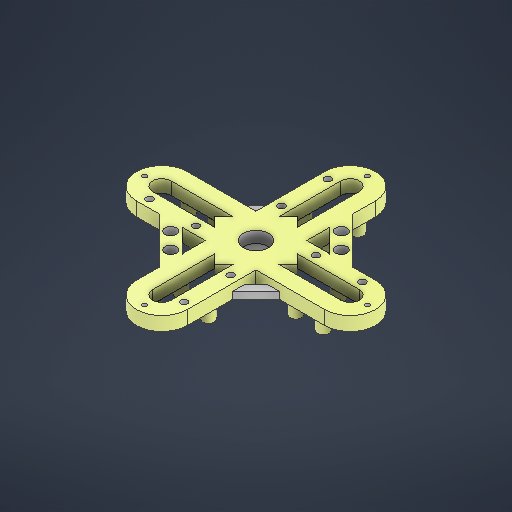
# Autodesk Inventor part: Redesign_Gripper_Baseplate
Saved by Autodesk Inventor 2025.1 (Build 291241000, 241)
## iProperties
Created: 2024-12-19
Part Number: Redesign_Gripper_Baseplate
Material: Generic
Document SubType Name: Modeling
Designer: m_kni
Density: 1 g/cm^3
Appearance: Default
Finish1_Area: 11299.045 mm^2
Finish1_Appearance: Satin - Lemon Chiffon
Finish1_Process: Prime/Paint RAL 3018
Finish1_Description: Prime/Paint RAL 3018
Finish1_ShortDescription: RAL 3018
Finish1_Thickness: 0.050 mm
Author: m_kni
## iProperties of the stored document Redesign_Gripper_Baseplate_3DPrint.ipt
Created: 2025-01-24
Part Number: Redesign_Gripper_Baseplate_3DPrint
Material: Generic
Document SubType Name: Modeling
Designer: m_kni
Density: 1 g/cm^3
Appearance: Default
Author: m_kni
Autodesk Inventor part; units mm, degrees
ref_plane "YZ Plane" through (0, 0, 0) normal (1, 0, 0) x (0, 1, 0)
ref_plane "XZ Plane" through (0, 0, 0) normal (0, 1, 0) x (-1, 0, 0)
ref_plane "XY Plane" through (0, 0, 0) normal (0, 0, 1) x (1, 0, 0)
sketch "Sketch1" plane through (0, 0, 0) normal (0, 1, 0) x (-1, 0, 0)
  line L0 (17.9605, 0) -> (0, -17.9605)
  line L1 (17.9605, 0) -> (43.3605, 0) construction
  line L2 (17.9605, 0) -> (0, 17.9605)
  line L3 (17.9605, 0) -> (43.3605, 0) construction
  line L4 (-17.9605, 0) -> (0, -17.9605)
  line L5 (-17.9605, 0) -> (0, 17.9605)
  line L6 (0, 15.4205) -> (-15.4205, 0)
  line L7 (0, 15.4205) -> (21.8079, 15.4205) construction
  line L8 (-15.4205, 0) -> (0, -15.4205)
  line L9 (0, -15.4205) -> (15.4205, 0)
  line L10 (15.4205, 0) -> (0, 15.4205)
  line L11 (0, -40.8205) -> (2, -40.8205)
  line L12 (0, -40.8205) -> (-2, -40.8205)
  circle A0 centre (7.5, -28.1205) radius 2.5
  line L13 (4, -28.1205) -> (4, -13.9605)
  line L14 (4, -28.1205) -> (4, -40.8205)
  line L15 (11, -6.9605) -> (11, -40.8205)
  arc A1 (-4, -40.8205) -> (4, -40.8205) centre (0, -40.8205) ccw
  line L16 (0, -15.4205) -> (0, -17.9605)
  line L17 (-4, -40.8205) -> (-4, -13.9605)
  line L18 (-11, -40.8205) -> (-11, -6.9605)
  arc A2 (-11, -40.8205) -> (11, -40.8205) centre (0, -40.8205) ccw
  circle A3 centre (-7.5, -24.8705) radius 2.5
  circle A4 centre (-7.5, -36.6205) radius 2.5
  line L19 (15.4205, 0) -> (17.9605, 0)
  line L20 (28.1205, 4) -> (13.9605, 4)
  circle A5 centre (28.1205, 7.5) radius 2.5
  circle A6 centre (24.8705, -7.5) radius 2.5
  line L21 (6.9605, 11) -> (40.8205, 11)
  line L22 (40.8205, -11) -> (6.9605, -11)
  line L23 (40.8205, -4) -> (13.9605, -4)
  line L24 (28.1205, 4) -> (40.8205, 4)
  line L25 (40.8205, 0) -> (40.8205, 2)
  circle A7 centre (36.6205, -7.5) radius 2.5
  line L26 (40.8205, 0) -> (40.8205, -2)
  arc A8 (40.8205, -4) -> (40.8205, 4) centre (40.8205, 0) ccw
  arc A9 (40.8205, -11) -> (40.8205, 11) centre (40.8205, 0) ccw
  line L27 (0, 15.4205) -> (0, 17.9605)
  line L28 (-4, 28.1205) -> (-4, 13.9605)
  circle A10 centre (-7.5, 28.1205) radius 2.5
  circle A11 centre (7.5, 24.8705) radius 2.5
  line L29 (-11, 6.9605) -> (-11, 40.8205)
  line L30 (11, 40.8205) -> (11, 6.9605)
  line L31 (4, 40.8205) -> (4, 13.9605)
  line L32 (-4, 28.1205) -> (-4, 40.8205)
  line L33 (0, 40.8205) -> (-2, 40.8205)
  circle A12 centre (7.5, 36.6205) radius 2.5
  line L34 (0, 40.8205) -> (2, 40.8205)
  arc A13 (4, 40.8205) -> (-4, 40.8205) centre (0, 40.8205) ccw
  arc A14 (11, 40.8205) -> (-11, 40.8205) centre (0, 40.8205) ccw
  line L35 (-15.4205, 0) -> (-17.9605, 0)
  line L36 (-28.1205, -4) -> (-13.9605, -4)
  circle A15 centre (-28.1205, -7.5) radius 2.5
  circle A16 centre (-24.8705, 7.5) radius 2.5
  line L37 (-6.9605, -11) -> (-40.8205, -11)
  line L38 (-40.8205, 11) -> (-6.9605, 11)
  line L39 (-40.8205, 4) -> (-13.9605, 4)
  line L40 (-28.1205, -4) -> (-40.8205, -4)
  line L41 (-40.8205, 0) -> (-40.8205, -2)
  circle A17 centre (-36.6205, 7.5) radius 2.5
  line L42 (-40.8205, 0) -> (-40.8205, 2)
  arc A18 (-40.8205, 4) -> (-40.8205, -4) centre (-40.8205, 0) ccw
  arc A19 (-40.8205, 11) -> (-40.8205, -11) centre (-40.8205, 0) ccw
  point P0 (0, 0)
  point P1 (0, -28.1205)
  point P2 (2, -28.1205)
  point P3 (-2, -22.1205)
  point P4 (-7.5, -22.1205)
  point P5 (-2, -34.1205)
  point P6 (-7.5, -34.1205)
  point P7 (11, -28.1205)
  point P8 (28.1205, 2)
  point P9 (28.1205, 11)
  point P10 (34.1205, -7.5)
  point P11 (34.1205, -2)
  point P12 (22.1205, -7.5)
  point P13 (22.1205, -2)
  point P14 (28.1205, 0)
  point P15 (-2, 28.1205)
  point P16 (-11, 28.1205)
  point P17 (7.5, 34.1205)
  point P18 (2, 34.1205)
  point P19 (7.5, 22.1205)
  point P20 (2, 22.1205)
  point P21 (0, 28.1205)
  point P22 (-28.1205, -2)
  point P23 (-28.1205, -11)
  point P24 (-34.1205, 7.5)
  point P25 (-34.1205, 2)
  point P26 (-22.1205, 7.5)
  point P27 (-22.1205, 2)
  point P28 (-28.1205, 0)
  point P29 (11, 11)
  point P30 (-11, 11)
  point P31 (-11, -11)
  point P32 (11, -11)
  dimension "d12" = 25.4
  dimension "d15" = 25.4
  dimension "d18" = 2.54
  dimension "d19" = 135
  dimension "d25" = 5
  dimension "d41" = 360
  constraints: 86 end point, 20 centre point, 16 coincident, 16 point on circle, 12 point on line, 5 vertical, 4 parallel, 3 equal length, 3 horizontal, 3 perpendicular, 173 other
  measures "d12" distance of L0.start L0.end
  measures "d15" distance of L0.start L2.end
  measures "d18" distance of L6.start L2.end
  measures "d19" angle of L6 L7
  measures "d25" diameter of A0
extrude "Extrusion1" add sketch "Sketch1" along normal blind 6 contours L19 L10 L27 L2 | L0 L16 L9 L19 | L23 A8 L24 L20 L2 L30 L21 A9 L22 L15 L0 | L9 L8 L6 L10 | L15 L22 L0 | L2 L21 L30 | L16 L4 L35 L8 | L6 L35 L5 L27 | L22 L15 A2 L18 L37 L4 L17 A1 L14 L13 L0 | L2 L31 A13 L32 L28 L5 L38 L29 A14 L30 L21 | L4 L18 L37 A19 L38 L29 L5 L39 A18 L40 L36 | L37 L18 L4 | L5 L29 L38 | A0 | A3 | A4 | A5 | A6 | A7 | A10 | A11 | A12 | A15 | A16 | A17
extrude "Extrusion2" add sketch "Sketch1" against normal blind 5.6 contours A0 | A3 | A4 | A5 | A6 | A7 | A10 | A11 | A12 | A15 | A16 | A17
sketch "Sketch2" plane through (0, 0, 0) normal (0, -1, 0) x (1, 0, 0)
  circle A0 centre (7.5, 28.1205) radius 2.5 projected
  circle A1 centre (7.5, 28.1205) radius 2.625
  circle A2 centre (-7.5, 36.6205) radius 2.5 projected
  circle A3 centre (-7.5, 36.6205) radius 2.625
  circle A4 centre (-7.5, 24.8705) radius 2.5 projected
  circle A5 centre (-7.5, 24.8705) radius 2.625
  circle A6 centre (-28.1205, 7.5) radius 2.625
  circle A7 centre (-36.6205, -7.5) radius 2.625
  circle A8 centre (-24.8705, -7.5) radius 2.625
  circle A9 centre (-7.5, -28.1205) radius 2.625
  circle A10 centre (7.5, -36.6205) radius 2.625
  circle A11 centre (7.5, -24.8705) radius 2.625
  circle A12 centre (28.1205, -7.5) radius 2.625
  circle A13 centre (36.6205, 7.5) radius 2.625
  circle A14 centre (24.8705, 7.5) radius 2.625
  point P0 (0, 0)
  dimension "d47" = 5.25
  dimension "d48" = 5.25
  dimension "d49" = 5.25
  dimension "d52" = 360
  constraints: 12 centre point, 3 coincident, 25 other
  measures "d47" diameter of A1
  measures "d48" diameter of A3
  measures "d49" diameter of A5
extrude "Extrusion3" add sketch "Sketch2" along normal blind 0.6 contours A0 | A1 | A2 | A3 | A4 | A5 | A6 | A7 | A8 | A9 | A10 | A11 | A12 | A13 | A14
sketch "Sketch3" plane through (7.5, -5.6, 28.1205) normal (0, -1, 0) x (1, 0, 0)
  circle A0 centre (0, 0) radius 1
  circle A1 centre (-15, 8.5) radius 2.5 projected
  circle A2 centre (-15, 8.5) radius 1
  circle A3 centre (-15, -3.25) radius 2.5 projected
  circle A4 centre (-15, -3.25) radius 1
  circle A5 centre (-44.1205, -35.6205) radius 1
  circle A6 centre (-32.3705, -35.6205) radius 1
  circle A7 centre (-35.6205, -20.6205) radius 1
  circle A8 centre (0, -64.741) radius 1
  circle A9 centre (0, -52.991) radius 1
  circle A10 centre (-15, -56.241) radius 1
  circle A11 centre (29.1205, -20.6205) radius 1
  circle A12 centre (17.3705, -20.6205) radius 1
  circle A13 centre (20.6205, -35.6205) radius 1
  point P0 (-7.5, -28.1205)
  dimension "d56" = 2
  dimension "d57" = 2
  dimension "d58" = 2
  dimension "d61" = 360
  constraints: 12 centre point, 2 coincident, 25 other
  measures "d56" diameter of A0
  measures "d57" diameter of A2
  measures "d58" diameter of A4
extrude "Extrusion4" cut sketch "Sketch3" against normal blind 6 contours A0 | A2 | A4 | A5 | A6 | A7 | A8 | A9 | A10 | A11 | A12 | A13
sketch "Sketch4" plane through (0, 6, 0) normal (0, 1, 0) x (1, 0, 0)
  circle A0 centre (0, 0) radius 5.5
  dimension "d65" = 11
  constraints: 1 centre point, 1 coincident
  measures "d65" diameter of A0
extrude "Extrusion5" cut sketch "Sketch4" against normal blind 5
ref_plane "Work Plane1" through (-40.8205, 0, 0) normal (0, 0, 1) x (1, 0, 0)
sketch "Sketch9" plane through (0, 0, 0) normal (0, -1, 0) x (1, 0, 0)
  circle A0 centre (-38.6205, 7.5) radius 1.5
  line L0 (0, 0) -> (7.5, 7.5)
  line L1 (0, 0) -> (10.6066, 0) construction
  circle A1 centre (38.6205, -7.5) radius 1.5
  circle A2 centre (28.1205, -7.5) radius 1 projected
  line L2 (0, 0) -> (0, 15)
  circle A3 centre (7.5, 38.6205) radius 1.5
  circle A4 centre (-38.6205, 7.5) radius 1.5
  circle A5 centre (-7.5, -38.6205) radius 1.5
  point P0 (-36.6205, -7.5)
  point P1 (-28.1205, 7.5)
  dimension "d83" = 3
  dimension "d84" = 10.5
  dimension "d87" = 45
  dimension "d88" = 3
  dimension "d89" = 10.5
  dimension "d96" = 360
  constraints: 6 end point, 5 centre point, 1 coincident, 1 equal length, 1 horizontal, 1 vertical, 9 other
  measures "d83" diameter of A0
  measures "d84" distance of point (-28.121, 7.5) A0.centre
  measures "d87" angle of L1 L0
  measures "d88" diameter of A1
  measures "d89" distance of A1.centre A2.centre
sketch "Sketch10" plane through (0, 6, 0) normal (0, 1, 0) x (1, 0, 0)
  line L0 (-11, 11) -> (-40.8205, 11) projected
  line L1 (-11, 11) -> (-16, 11)
  line L2 (-16, 11) -> (-16, 16)
  line L3 (-16, 16) -> (-11, 16)
  line L4 (-11, 16) -> (-11, 11)
  line L5 (-11, 16) -> (-16, 11)
  line L6 (-16, 16) -> (-21, 11)
  line L7 (-16, 16) -> (-11, 21)
  line L8 (-11, 40.8205) -> (-11, 11) projected
  line L9 (40.8205, 11) -> (11, 11) projected
  line L10 (11, 11) -> (-11, -11)
  line L11 (11, -11) -> (11, -16)
  line L12 (11, -16) -> (16, -16)
  line L13 (16, -16) -> (16, -11)
  line L14 (16, -11) -> (11, -11)
  line L15 (16, -11) -> (11, -16)
  line L16 (16, -16) -> (11, -21)
  line L17 (16, -16) -> (21, -11)
  line L18 (11, -11) -> (40.8205, -11) projected
  line L19 (21, -11) -> (11, -11)
  line L20 (11, -11) -> (11, -21)
  point P0 (0, 0)
  dimension "d90" = 5
  dimension "d91" = 5
  constraints: 34 end point, 6 symmetric about line, 4 point on line, 3 perpendicular, 2 parallel, 1 horizontal
  measures "d90" distance of L2.end L3.end
  measures "d91" distance of L1.end L2.end
extrude "Extrusion11" add sketch "Sketch10" against normal up to surface (6 mm away) contours L0 L6 L2 | L2 L3 L5 | L3 L7 L8 | L15 L13 L12 | L12 L16 L20 | L18 L17 L13
extrude "Extrusion12" cut sketch "Sketch9" against normal up to surface (6 mm away) contours A0 | A1 | A3 | A5
sketch "Sketch11" plane through (0, 6, 0) normal (0, 1, 0) x (1, 0, 0)
  line L0 (-40.8205, -11) -> (-11, -11) projected
  line L1 (-11, -11) -> (-21, -11)
  line L2 (-21, -11) -> (-21, -21)
  line L3 (-21, -21) -> (-11, -21)
  line L4 (-11, -21) -> (-11, -11)
  line L5 (11, 11) -> (11, 40.8205) projected
  line L6 (11, 11) -> (21, 11)
  line L7 (21, 11) -> (21, 21)
  line L8 (21, 21) -> (11, 21)
  line L9 (11, 21) -> (11, 11)
  line L10 (11, 11) -> (31, 11)
  line L11 (11, 31) -> (11, 11)
  line L12 (-11, -11) -> (-31, -11)
  line L13 (-11, -31) -> (-11, -11)
  line L14 (-11, -21) -> (-21, -11)
  line L15 (-11, -31) -> (-31, -11)
  line L16 (21, 11) -> (11, 21)
  line L17 (31, 11) -> (11, 31)
  line L18 (-11, -11) -> (-11, -40.8205) projected
  point P0 (0, 0)
  dimension "d100" = 10
  dimension "d101" = 10
  dimension "d102" = 10
  dimension "d103" = 10
  constraints: 32 end point, 5 parallel, 4 horizontal, 2 perpendicular
  measures "d100" distance of L3.end L2.end
  measures "d101" distance of L2.end L1.end
  measures "d102" distance of L8.end L7.end
  measures "d103" distance of L7.end L6.end
extrude "Extrusion13" add sketch "Sketch11" against normal up to surface (6 mm away) contours L0 L2 L15 | L14 L3 L2 | L3 L13 L15 | L5 L17 L8 | L8 L7 L16 | L7 L17 L10
sketch "Sketch12" plane through (0, 6, 0) normal (0, 1, 0) x (1, 0, 0)
  line L0 (-31, -11) -> (-11, -31) projected
  line L1 (-11, -21) -> (-21, -11) projected
  line L2 (11, 21) -> (21, 11) projected
  line L3 (31, 11) -> (11, 31) projected
  line L4 (-11, -31) -> (-11, -21)
  line L5 (-21, -11) -> (-31, -11)
  line L6 (11, 21) -> (11, 31)
  line L7 (21, 11) -> (11, 11) projected
  line L8 (21, 11) -> (31, 11)
  line L9 (26, 11) -> (11, 26)
  line L10 (-11, -26) -> (-26, -11)
  line L11 (-16, -16) -> (-21, -21)
  line L12 (16, 16) -> (21, 21)
  circle A0 centre (-14.9645, -22.0355) radius 2.5
  circle A1 centre (-22.0355, -14.9645) radius 2.5
  circle A2 centre (22.0355, 14.9645) radius 2.5
  circle A3 centre (14.9645, 22.0355) radius 2.5
  point P0 (0, 0)
  dimension "d110" = 5
  dimension "d111" = 5
  dimension "d112" = 5
  dimension "d113" = 5
  dimension "d114" = 5
  dimension "d115" = 5
  dimension "d116" = 5
  dimension "d117" = 5
  constraints: 16 end point, 8 midpoint, 4 centre point, 4 point on line, 3 perpendicular, 1 vertical
  measures "d110" diameter of A0
  measures "d111" distance from line of L11 A0.centre
  measures "d112" distance from line of L11 A1.centre
  measures "d113" diameter of A1
  measures "d114" diameter of A2
  measures "d115" diameter of A3
  measures "d116" distance from line of A3.centre L12
  measures "d117" distance from line of L12 A2.centre
extrude "Extrusion14" cut sketch "Sketch12" against normal up to surface (6 mm away) contours A1 L10 | L10 A1 | A0 L10 | L10 A0 | A3 L9 | L9 A3 | A2 L9 | L9 A2
sketch "Sketch13" plane through (0, 6, 0) normal (0, 1, 0) x (1, 0, 0)
  line L0 (21, -11) -> (40.8205, -11) projected
  line L1 (11, -11) -> (16, -11) projected
  line L2 (21, -11) -> (16, -11)
  line L3 (11, -16) -> (11, -11) projected
  line L4 (16, -11) -> (11, -16)
  line L5 (11, -21) -> (21, -11) projected
  line L6 (21, -11) -> (11, -21)
  line L7 (11, -21) -> (11, -16)
  line L8 (-11, 16) -> (-16, 11)
  line L9 (-16, 11) -> (-21, 11)
  line L10 (-21, 11) -> (-11, 21)
  line L11 (-11, 21) -> (-11, 16)
  point P0 (0, 0)
  constraints: 16 end point, 2 parallel, 2 perpendicular, 1 collinear, 1 horizontal, 1 vertical
extrude "Extrusion15" cut sketch "Sketch13" against normal blind 3 contours L2 L5 L7 L4 | L8 L9 L10 L11
sketch "Sketch14" plane through (0, 0, 0) normal (0, -1, 0) x (1, 0, 0)
  arc A0 (11, 40.8205) -> (-11, 40.8205) centre (0, 40.8205) ccw projected
  arc A1 (4, 40.8205) -> (-4, 40.8205) centre (0, 40.8205) ccw projected
  line L0 (0, 51.8205) -> (0, 44.8205)
  circle A2 centre (0, 48.3205) radius 1
  circle A3 centre (-48.3205, 0) radius 1
  circle A4 centre (0, -48.3205) radius 1
  circle A5 centre (48.3205, 0) radius 1
  point P0 (0, 0)
  dimension "d122" = 2
  dimension "d125" = 360
  constraints: 4 centre point, 2 end point, 2 point on circle, 1 coincident, 1 midpoint, 1 vertical, 9 other
  measures "d122" diameter of A2
extrude "Extrusion16" cut sketch "Sketch14" against normal blind 10
fillet "Fillet1" radius 0.5 12 edges at (-4, 0, 27.3905) (4, 0, 27.3905) (0, 0, 44.8205) (-27.3905, 0, -4) (-27.3905, 0, 4) (-44.8205, 0, 0) (44.8205, 0, 0) (27.3905, 0, 4) (27.3905, 0, -4) (0, 0, -44.8205) (-4, 0, -27.3905) (4, 0, -27.3905) curvature continuous yes
sketch "Sketch15" plane through (0, 6, 0) normal (0, 1, 0) x (1, 0, 0)
  line L0 (21, -11) -> (11, -21) projected
  line L1 (11, -16) -> (16, -11) projected
  line L2 (11, -40.8205) -> (11, -11) projected
  line L3 (11, -16) -> (11, -21)
  line L4 (11, -18.5) -> (4, -18.5)
  line L5 (4, -13.9605) -> (4, -40.8205) projected
  circle A0 centre (7.5, -18.5) radius 1.5
  circle A1 centre (18.5, 7.5) radius 1.5
  circle A2 centre (-7.5, 18.5) radius 1.5
  circle A3 centre (-18.5, -7.5) radius 1.5
  point P0 (0, 0)
  dimension "d130" = 3
  dimension "d133" = 360
  constraints: 4 centre point, 4 end point, 2 midpoint, 1 coincident, 1 perpendicular, 1 point on line, 1 vertical, 9 other
  measures "d130" diameter of A0
extrude "Extrusion17" cut sketch "Sketch15" against normal blind 10
equation "\"d92\" = d91"
equation "\"d108\" = d103"
body "Solid1"
